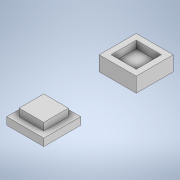
# Autodesk Inventor part: InsertTest
Saved by Autodesk Inventor 2022 (Build 260153000, 153)
## iProperties
Created: 2022-04-20
Part Number: InsertTest
Material: Generic
Document SubType Name: Modeling
Designer: Bruger
Density: 1 g/cm^3
Appearance: Default
Author: Bruger
Autodesk Inventor part; units mm, degrees
ref_plane "YZ Plane" through (0, 0, 0) normal (1, 0, 0) x (0, 1, 0)
ref_plane "XZ Plane" through (0, 0, 0) normal (0, 1, 0) x (-1, 0, 0)
ref_plane "XY Plane" through (0, 0, 0) normal (0, 0, 1) x (1, 0, 0)
sketch "Sketch1" plane through (0, 0, 0) normal (0, 1, 0) x (-1, 0, 0)
  line L0 (-7.5, 7.5) -> (7.5, 7.5)
  line L1 (7.5, 7.5) -> (7.5, -7.5)
  line L2 (7.5, -7.5) -> (-7.5, -7.5)
  line L3 (-7.5, -7.5) -> (-7.5, 7.5)
  line L4 (-7.5, 7.5) -> (7.5, -7.5) construction
  line L5 (7.5, 7.5) -> (-7.5, -7.5) construction
  line L6 (-5, 5) -> (5, 5)
  line L7 (5, 5) -> (5, -5)
  line L8 (5, -5) -> (-5, -5)
  line L9 (-5, -5) -> (-5, 5)
  line L10 (-5, 5) -> (5, -5) construction
  line L11 (5, 5) -> (-5, -5) construction
  line L12 (0, -7.5) -> (0, -37.5)
  line L13 (-7.5, -45) -> (7.5, -45)
  line L14 (7.5, -45) -> (7.5, -30)
  line L15 (7.5, -30) -> (-7.5, -30)
  line L16 (-7.5, -30) -> (-7.5, -45)
  line L17 (-7.5, -45) -> (7.5, -30) construction
  line L18 (7.5, -45) -> (-7.5, -30) construction
  line L19 (-5.1, -42.6) -> (5.1, -42.6)
  line L20 (5.1, -42.6) -> (5.1, -32.4)
  line L21 (5.1, -32.4) -> (-5.1, -32.4)
  line L22 (-5.1, -32.4) -> (-5.1, -42.6)
  line L23 (-5.1, -42.6) -> (5.1, -32.4) construction
  line L24 (5.1, -42.6) -> (-5.1, -32.4) construction
  point P0 (0, 0)
  dimension "d0" = 15
  dimension "d1" = 15
  dimension "d2" = 10
  dimension "d3" = 10
  dimension "d4" = 30
  dimension "d5" = 15
  dimension "d6" = 15
  dimension "d7" = 10.2
  dimension "d8" = 10.2
  constraints: 50 end point, 9 midpoint, 8 parallel, 4 horizontal, 4 perpendicular, 1 vertical
  measures "d0" distance of L1.end L2.end
  measures "d1" distance of L0.end L1.end
  measures "d2" distance of L7.end L8.end
  measures "d3" distance of L6.end L7.end
  measures "d4" distance of L12.start L12.end
  measures "d5" distance of L15.end L14.end
  measures "d6" distance of L14.end L13.end
  measures "d7" distance of L21.end L20.end
  measures "d8" distance of L20.end L19.end
extrude "Extrusion3" add sketch "Sketch1" along normal blind 3 contours L0 L1 L2 L3
extrude "Extrusion4" add sketch "Sketch1" along normal blind 6 contours L6 L7 L8 L9
extrude "Extrusion5" add sketch "Sketch1" along normal blind 6 contours L15 L14 L13 L16
extrude "Extrusion6" add sketch "Sketch1" along normal blind 3 contours L21 L20 L19 L22
body "Solid2"
